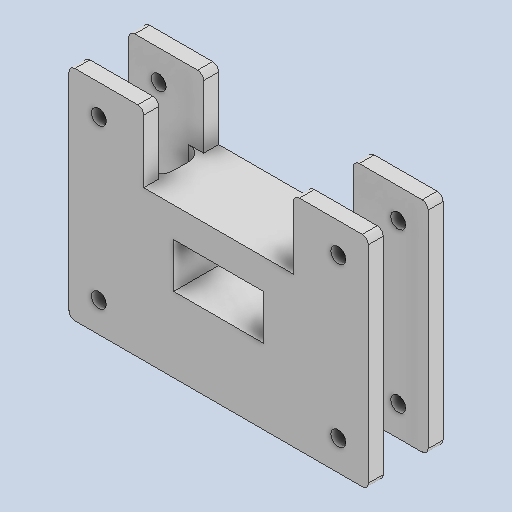
# Autodesk Inventor part: BracketPenghubung
Saved by Autodesk Inventor 2026.2 (Build 302298010, 298A)
## iProperties
Created: 2026-05-29
Part Number: BracketPenghubung
Material: Generic
Document SubType Name: Modeling
Designer: rizky
Density: 1 g/cm^3
Appearance: Default
Author: rizky
Autodesk Inventor part; units mm, degrees
ref_plane "YZ Plane" through (0, 0, 0) normal (1, 0, 0) x (0, 1, 0)
ref_plane "XZ Plane" through (0, 0, 0) normal (0, 1, 0) x (-1, 0, 0)
ref_plane "XY Plane" through (0, 0, 0) normal (0, 0, 1) x (1, 0, 0)
sketch "Sketch1" plane through (0, 0, 0) normal (0, 0, 1) x (1, 0, 0)
  line L0 (0, 0) -> (100, 0)
  line L1 (100, 0) -> (100, 73)
  line L2 (100, 73) -> (0, 73)
  line L3 (0, 73) -> (0, 0)
  line L4 (0, 73) -> (10, 73)
  line L5 (10, 73) -> (10, 63)
  circle A0 centre (10, 63) radius 2.5
  line L6 (50, 73) -> (50, 68)
  line L7 (0, 36.5) -> (5, 36.5)
  circle A1 centre (90, 63) radius 2.5
  circle A2 centre (10, 10) radius 2.5
  circle A3 centre (90, 10) radius 2.5
  line L8 (50, 0) -> (50, 25)
  line L9 (50, 25) -> (65, 25)
  line L10 (65, 25) -> (65, 40)
  line L11 (65, 40) -> (50, 40)
  line L12 (50, 40) -> (50, 25)
  line L13 (50, 25) -> (35, 25)
  line L14 (35, 25) -> (35, 40)
  line L15 (35, 40) -> (50, 40)
  dimension "d0" = 100
  dimension "d1" = 73
  dimension "d2" = 10
  dimension "d3" = 10
  dimension "d4" = 5
  dimension "d5" = 5
  dimension "d6" = 5
  dimension "d7" = 25
  dimension "d8" = 15
  dimension "d9" = 15
  constraints: 32 end point, 5 symmetric about line, 4 centre point, 4 parallel, 3 horizontal, 3 midpoint, 3 perpendicular, 2 vertical, 1 coincident, 1 point on line, 3 other
  measures "d0" distance of L2.end L1.end
  measures "d1" distance of L1.end L0.end
  measures "d2" distance of L2.end L4.end
  measures "d3" distance of L4.end L5.end
  measures "d4" diameter of A0
  measures "d5" distance of L6.start L6.end
  measures "d6" distance of L7.start L7.end
  measures "d7" distance of L8.start L8.end
  measures "d8" distance of L11.end L10.end
  measures "d9" distance of L10.end L9.end
extrude "Extrusion1" add sketch "Sketch1" along normal blind 5
sketch "Sketch2" plane through (0, 0, 5) normal (0, 0, 1) x (1, 0, 0)
  line L0 (100, 0) -> (100, 73) projected
  line L1 (100, 73) -> (0, 73) projected
  line L2 (0, 73) -> (0, 0) projected
  line L3 (0, 0) -> (100, 0) projected
  line L4 (65, 25) -> (35, 25) projected
  line L5 (35, 25) -> (35, 40) projected
  line L6 (35, 40) -> (65, 40) projected
  line L7 (65, 40) -> (65, 25) projected
  circle A0 centre (10, 63) radius 2.5 projected
  circle A1 centre (90, 63) radius 2.5 projected
  circle A2 centre (10, 10) radius 2.5 projected
  circle A3 centre (90, 10) radius 2.5 projected
  line L8 (75, 50) -> (25, 50)
  line L9 (25, 50) -> (25, 15)
  line L10 (25, 15) -> (75, 15)
  line L11 (75, 15) -> (75, 50)
  line L12 (25, 50) -> (25, 73)
  line L13 (25, 15) -> (25, 0)
  line L14 (50, 50) -> (50, 40)
  line L15 (75, 50) -> (75, 73)
  line L16 (75, 15) -> (75, 0)
  dimension "d12" = 10
  dimension "d13" = 10
  constraints: 18 end point, 2 perpendicular, 2 point on line, 2 symmetric about line, 1 midpoint, 1 vertical, 3 other
  measures "d12" distance between parallel lines of L6 L8
  measures "d13" distance of L14.start L14.end
extrude "Extrusion2" cut sketch "Sketch2" against normal blind 5 contours L3 L13 L10 L16 | L15 L8 L12 L1
sketch "Sketch3" plane through (0, 0, 5) normal (0, 0, 1) x (1, 0, 0)
  line L0 (75, 15) -> (75, 0) projected
  line L1 (75, 0) -> (100, 0) projected
  line L2 (100, 0) -> (100, 73) projected
  line L3 (100, 73) -> (75, 73) projected
  line L4 (75, 73) -> (75, 50) projected
  line L5 (75, 50) -> (25, 50) projected
  line L6 (25, 50) -> (25, 73) projected
  line L7 (25, 73) -> (0, 73) projected
  line L8 (0, 73) -> (0, 0) projected
  line L9 (0, 0) -> (25, 0) projected
  line L10 (25, 0) -> (25, 15) projected
  line L11 (25, 15) -> (75, 15) projected
  line L12 (65, 25) -> (35, 25) projected
  line L13 (35, 25) -> (35, 40) projected
  line L14 (35, 40) -> (65, 40) projected
  line L15 (65, 40) -> (65, 25) projected
  circle A0 centre (10, 63) radius 2.5 projected
  circle A1 centre (90, 63) radius 2.5 projected
  circle A2 centre (10, 10) radius 2.5 projected
  circle A3 centre (90, 10) radius 2.5 projected
  line L16 (25, 50) -> (25, 15)
  line L17 (75, 50) -> (75, 15)
  constraints: 4 end point, 1 parallel, 1 vertical
extrude "Extrusion3" add sketch "Sketch3" along normal blind 20 contours L11 L16 L5 L17
sketch "Sketch4" plane through (0, 0, 25) normal (0, 0, 1) x (1, 0, 0)
  circle A0 centre (90, 10) radius 2.5 projected
  circle A1 centre (90, 63) radius 2.5 projected
  line L0 (75, 50) -> (75, 15) projected
  line L1 (75, 15) -> (75, 0) projected
  line L2 (75, 0) -> (100, 0) projected
  line L3 (100, 0) -> (100, 73) projected
  line L4 (100, 73) -> (75, 73) projected
  line L5 (75, 73) -> (75, 50) projected
  line L6 (25, 15) -> (25, 50) projected
  line L7 (25, 50) -> (25, 73) projected
  line L8 (25, 73) -> (0, 73) projected
  line L9 (0, 73) -> (0, 0) projected
  line L10 (0, 0) -> (25, 0) projected
  line L11 (25, 0) -> (25, 15) projected
  circle A2 centre (10, 63) radius 2.5 projected
  circle A3 centre (10, 10) radius 2.5 projected
extrude "Extrusion4" add sketch "Sketch4" against normal blind 5
fillet "Fillet1" radius 2 12 edges at (0, 73, 2.5) (100, 73, 2.5) (75, 73, 2.5) (25, 73, 2.5) (25, 73, 22.5) (75, 73, 22.5) (100, 73, 22.5) (0, 73, 22.5) (0, 0, 22.5) (0, 0, 2.5) (100, 0, 2.5) (100, 0, 22.5)
sketch "Sketch5" plane through (0, 0, 25) normal (0, 0, 1) x (1, 0, 0)
  arc A0 (98, 0) -> (100, 2) centre (98, 2) ccw projected
  line L0 (100, 2) -> (100, 71) projected
  arc A1 (100, 71) -> (98, 73) centre (98, 71) ccw projected
  line L1 (98, 73) -> (77, 73) projected
  arc A2 (77, 73) -> (75, 71) centre (77, 71) ccw projected
  line L2 (75, 71) -> (75, 50) projected
  line L3 (75, 50) -> (25, 50) projected
  line L4 (25, 50) -> (25, 71) projected
  arc A3 (25, 71) -> (23, 73) centre (23, 71) ccw projected
  line L5 (23, 73) -> (2, 73) projected
  arc A4 (2, 73) -> (0, 71) centre (2, 71) ccw projected
  line L6 (0, 71) -> (0, 2) projected
  arc A5 (0, 2) -> (2, 0) centre (2, 2) ccw projected
  line L7 (2, 0) -> (25, 0) projected
  line L8 (25, 0) -> (25, 15) projected
  line L9 (25, 15) -> (75, 15) projected
  line L10 (75, 15) -> (75, 0) projected
  line L11 (75, 0) -> (98, 0) projected
  circle A6 centre (90, 63) radius 2.5 projected
  circle A7 centre (90, 10) radius 2.5 projected
  circle A8 centre (10, 10) radius 2.5 projected
  circle A9 centre (10, 63) radius 2.5 projected
  line L12 (65, 25) -> (35, 25) projected
  line L13 (35, 25) -> (35, 40) projected
  line L14 (35, 40) -> (65, 40) projected
  line L15 (65, 40) -> (65, 25) projected
  line L16 (25, 0) -> (75, 0)
  point P0 (0, 0)
  constraints: 2 end point, 1 horizontal
extrude "Extrusion5" add sketch "Sketch5" against normal blind 5 contours L16 L8 L9 L10
sketch "Sketch6" plane through (0, 0, 0) normal (0, 0, -1) x (-1, 0, 0)
  arc A0 (-100, 2) -> (-98, 0) centre (-98, 2) ccw projected
  line L0 (-75, 0) -> (-98, 0) projected
  line L1 (-75, 0) -> (-75, 15) projected
  line L2 (-75, 15) -> (-25, 15) projected
  line L3 (-25, 15) -> (-25, 0) projected
  line L4 (-2, 0) -> (-25, 0) projected
  arc A1 (-2, 0) -> (0, 2) centre (-2, 2) ccw projected
  line L5 (0, 71) -> (0, 2) projected
  arc A2 (0, 71) -> (-2, 73) centre (-2, 71) ccw projected
  line L6 (-23, 73) -> (-2, 73) projected
  arc A3 (-23, 73) -> (-25, 71) centre (-23, 71) ccw projected
  line L7 (-25, 71) -> (-25, 50) projected
  line L8 (-25, 50) -> (-75, 50) projected
  line L9 (-75, 50) -> (-75, 71) projected
  arc A4 (-75, 71) -> (-77, 73) centre (-77, 71) ccw projected
  line L10 (-98, 73) -> (-77, 73) projected
  arc A5 (-98, 73) -> (-100, 71) centre (-98, 71) ccw projected
  line L11 (-100, 2) -> (-100, 71) projected
  circle A6 centre (-90, 10) radius 2.5 projected
  circle A7 centre (-10, 10) radius 2.5 projected
  circle A8 centre (-90, 63) radius 2.5 projected
  circle A9 centre (-10, 63) radius 2.5 projected
  line L12 (-65, 25) -> (-35, 25) projected
  line L13 (-65, 40) -> (-65, 25) projected
  line L14 (-35, 40) -> (-65, 40) projected
  line L15 (-35, 25) -> (-35, 40) projected
  line L16 (-25, 0) -> (-75, 0)
  point P0 (0, 0)
  constraints: 2 end point, 1 horizontal
extrude "Extrusion6" add sketch "Sketch6" against normal blind 5 contours L1 L2 L3 L16
move faces "Move1" translate (0, 5, 0) faces at (41.6667, 15, 10)
fillet "Fillet3" radius 5 4 edges at (25, 35, 5) (25, 35, 20) (75, 35, 5) (75, 35, 20)
body "Solid1"
